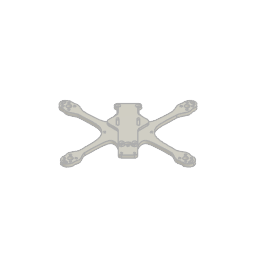
moineau (Autodesk Fusion 360 design; units mm, degrees)
Autodesk Fusion 360 part; units mm, degrees
sketch "Sketch1" plane through (0, 0, 0) normal (0, 0, 1) x (1, 0, 0)
  circle A0 centre (55.8574, 6.7392) radius 4.5 construction
  line L0 (55.8574, 6.7392) -> (52.6754, 9.9212) construction
  line L1 (219.6626, 222.0359) -> (219.6626, 222.0359)
  circle A1 centre (52.6754, 9.9212) radius 1.05
  circle A2 centre (55.8574, 6.7392) radius 2.25
  line L2 (42.8574, 9.2392) -> (42.8574, 4.2392) construction
  line L3 (55.8574, 6.7392) -> (61.4123, 6.7392) construction
  spline S0 degree 5 poles (64.6052, 6.7392) (64.6028, 6.815) (64.5921, 6.9823) (64.5587, 7.2805) (64.4799, 7.7571) (64.3247, 8.4054) (64.1108, 9.0216) (63.8323, 9.553) (63.4775, 10.0087) (63.0354, 10.4282) (62.4998, 10.855) (61.8755, 11.308) (61.1831, 11.7559) (60.4518, 12.1419) (59.713, 12.4068) (58.994, 12.5114) (58.3111, 12.462) (57.6641, 12.3267) (57.041, 12.1976) (56.421, 12.1615) (55.7776, 12.2677) (55.0823, 12.4938) (54.3087, 12.7668) (53.4369, 12.9885) (52.4575, 13.0608) (51.3775, 12.9063) (50.2215, 12.502) (49.011, 11.8911) (47.7686, 11.1568) (46.5151, 10.408) (45.2684, 9.7601) (44.2882, 9.4068) (43.567, 9.2696) (43.0928, 9.2392) (42.8574, 9.2392) knots 0 0 0 0 0 0 0.033333 0.066667 0.1 0.133333 0.166667 0.2 0.233333 0.266667 0.3 0.333333 0.366667 0.4 0.433333 0.466667 0.5 0.533333 0.566667 0.6 0.633333 0.666667 0.7 0.733333 0.766667 0.8 0.833333 0.866667 0.9 0.933333 0.966667 1 1 1 1 1 1
  line L4 (54.2959, 13.1912) -> (50.0454, 12.7812)
  line L5 (64.6536, 5.2576) -> (64.5569, 8.2208)
  line L6 (44.8576, 9.239) -> (40.8572, 9.2393)
  line L7 (0, 0) -> (70.7107, 70.7107) construction
  line L8 (-12.75, 12.75) -> (12.75, 12.75) construction
  line L9 (12.75, 12.75) -> (12.75, -12.75) construction
  line L10 (12.75, -12.75) -> (-12.75, -12.75) construction
  line L11 (-12.75, -12.75) -> (-12.75, 12.75) construction
  line L12 (12.75, -12.75) -> (-12.75, 12.75) construction
  circle A3 centre (12.75, 12.75) radius 1.05
  circle A4 centre (12.75, -12.75) radius 1.05
  line L13 (12.75, -12.75) -> (19.8211, -19.8211) construction
  line L14 (19.9636, -9.357) -> (25.1244, -14.5178)
  line L15 (12.75, 12.75) -> (14.9037, 12.0987) construction
  line L16 (12.75, 12.75) -> (15.3173, 13.1187) construction
  circle A5 centre (-12.75, 12.75) radius 1.05
  spline S1 degree 5 poles (60.9811, 6.7392) (60.9811, 6.886) (60.9796, 7.1794) (60.9724, 7.6186) (60.9623, 8.1894) (60.9925, 8.8095) (61.1129, 9.2564) (61.3477, 9.4734) (61.6899, 9.4412) (62.0445, 9.2424) (62.3497, 8.953) (62.5856, 8.6227) (62.7528, 8.2869) (62.8658, 7.964) (62.9398, 7.6579) (62.9854, 7.3611) (63.005, 7.1209) (63.0122, 6.9335) (63.0138, 6.8046) (63.0138, 6.7392) knots 0 0 0 0 0 0 0.066667 0.133333 0.2 0.266667 0.333333 0.4 0.466667 0.533333 0.6 0.666667 0.733333 0.8 0.866667 0.933333 1 1 1 1 1 1
  line L17 (60.9811, 5.9005) -> (60.9811, 7.5778)
  line L18 (61.2671, 9.4784) -> (61.9183, 9.3698)
  line L19 (63.0138, 7.3223) -> (63.0138, 6.1561)
  circle A6 centre (52.6754, 3.5572) radius 1.05
  circle A7 centre (59.0394, 3.5572) radius 1.05
  circle A8 centre (59.0394, 9.9212) radius 1.05
  circle A9 centre (23.3566, -16.2855) radius 1
  circle A10 centre (-12.75, 12.75) radius 1.05
  circle A11 centre (-12.75, 12.75) radius 1.05
  circle A12 centre (16.2855, -23.3566) radius 1
  circle A13 centre (12.75, -12.75) radius 1.05
  line L20 (9.357, -19.9636) -> (14.5178, -25.1244)
  line L21 (-12.75, 12.75) -> (-14.8713, 14.8713) construction
  line L22 (-20.3514, 9.3912) -> (-9.3912, 20.3514) construction
  circle A14 centre (-9.3912, 20.3514) radius 1.05
  circle A15 centre (-20.3514, 9.3912) radius 1.05
  line L23 (-19.114, 29.0135) -> (-29.0135, 19.114)
  line L24 (-12.75, 12.75) -> (-38.0129, 38.0129) construction
  line L25 (-19.114, 29.0135) -> (-17.1216, 29.1878)
  line L26 (-17.1216, 29.1878) -> (-11.2505, 23.3167)
  spline S2 degree 5 poles (-11.2505, 23.3167) (-11.2214, 23.2876) (-11.14, 23.2369) (-10.9486, 23.1834) (-10.5781, 23.1487) (-10.0185, 23.1302) (-9.5696, 23.1041) (-9.2669, 23.0627) (-9.0856, 23.0229) (-9, 23) knots 0 0 0 0 0 0 0.2 0.4 0.6 0.8 1 1 1 1 1 1
  line L27 (-11.5038, 23.57) -> (-10.9973, 23.0635)
  arc A16 (11.159, 11.1591) -> (11.1591, 11.1591) centre (10.8877, 13.3927) ccw
  arc A17 (-11.159, -11.1591) -> (-11.1591, -11.159) centre (-12.75, -12.75) ccw
  line L28 (-9.8162, 23.2188) -> (-8.1838, 22.7812)
  circle A18 centre (-12.75, -12.75) radius 1.05
  line L29 (-29.1878, 17.1216) -> (-23.3167, 11.2505)
  spline S3 degree 5 poles (-23.3167, 11.2505) (-23.2876, 11.2214) (-23.2369, 11.14) (-23.1834, 10.9486) (-23.1487, 10.5781) (-23.1302, 10.0185) (-23.1041, 9.5696) (-23.0627, 9.2669) (-23.0229, 9.0856) (-23, 9) knots 0 0 0 0 0 0 0.2 0.4 0.6 0.8 1 1 1 1 1 1
  line L30 (-23.57, 11.5038) -> (-23.0635, 10.9973)
  line L31 (-23.2188, 9.8162) -> (-22.7812, 8.1838)
  line L32 (-29.0135, 19.114) -> (-29.1878, 17.1216)
  line L33 (23.3566, -16.2855) -> (16.2855, -23.3566) construction
  line L34 (18.0533, -25.1244) -> (25.1244, -18.0533)
  arc A19 (14.5178, -25.1244) -> (18.0533, -25.1244) centre (16.2855, -23.3566) ccw
  arc A20 (18.0533, -21.5888) -> (17.6838, -21.2842) centre (16.2855, -23.3566) ccw construction
  arc A21 (21.2842, -17.6838) -> (21.5888, -18.0533) centre (23.3566, -16.2855) ccw construction
  arc A22 (25.1244, -18.0533) -> (25.1244, -14.5178) centre (23.3566, -16.2855) ccw
  line L35 (14.5345, -21.6048) -> (14.5054, -21.6339)
  line L36 (21.4731, -14.6417) -> (21.7061, -14.4078)
  circle A23 centre (55.8574, 6.7392) radius 37 construction
  spline S4 degree 5 poles (64.6052, 6.7392) (64.6028, 6.6634) (64.5921, 6.4961) (64.5587, 6.1979) (64.4799, 5.7213) (64.3247, 5.073) (64.1108, 4.4567) (63.8323, 3.9254) (63.4775, 3.4697) (63.0354, 3.0502) (62.4998, 2.6234) (61.8755, 2.1704) (61.1831, 1.7225) (60.4518, 1.3365) (59.713, 1.0715) (58.994, 0.967) (58.3111, 1.0163) (57.6641, 1.1517) (57.041, 1.2807) (56.421, 1.3168) (55.7776, 1.2106) (55.0823, 0.9846) (54.3087, 0.7116) (53.4369, 0.4899) (52.4575, 0.4175) (51.3775, 0.572) (50.2215, 0.9763) (49.011, 1.5872) (47.7686, 2.3215) (46.5151, 3.0704) (45.2684, 3.7183) (44.2882, 4.0715) (43.567, 4.2087) (43.0928, 4.2392) (42.8574, 4.2392) knots 0 0 0 0 0 0 0.033333 0.066667 0.1 0.133333 0.166667 0.2 0.233333 0.266667 0.3 0.333333 0.366667 0.4 0.433333 0.466667 0.5 0.533333 0.566667 0.6 0.633333 0.666667 0.7 0.733333 0.766667 0.8 0.833333 0.866667 0.9 0.933333 0.966667 1 1 1 1 1 1
  line L37 (64.6536, 8.2208) -> (64.5569, 5.2576)
  line L38 (54.2959, 0.2872) -> (50.0454, 0.6972)
  line L39 (44.8576, 4.2393) -> (40.8572, 4.239)
  circle A24 centre (55.8574, 6.7392) radius 34.5 construction
  circle A25 centre (12.75, 12.75) radius 2.25 construction
  spline S5 degree 5 poles (42.8574, 9.2392) (41.9558, 9.2392) (40.1768, 9.2381) (37.5805, 9.2331) (34.2689, 9.2281) (30.4157, 9.273) (26.8997, 9.4308) (23.7764, 9.7638) (21.0905, 10.3188) (18.8586, 11.1117) (17.0345, 12.0983) (15.8354, 12.979) (15.0487, 13.6574) (14.5694, 14.1126) (14.341, 14.341) knots 0 0 0 0 0 0 0.1 0.2 0.3 0.4 0.5 0.6 0.7 0.8 0.9 1 1 1 1 1 1
  line L40 (55.8574, 6.7392) -> (39.6365, 6.7392) construction
  spline S6 degree 5 poles (60.9811, 6.7392) (60.9811, 6.5924) (60.9796, 6.299) (60.9724, 5.8597) (60.9623, 5.2889) (60.9925, 4.6689) (61.1129, 4.2219) (61.3477, 4.005) (61.6899, 4.0372) (62.0445, 4.2359) (62.3497, 4.5254) (62.5856, 4.8556) (62.7528, 5.1915) (62.8658, 5.5144) (62.9398, 5.8204) (62.9854, 6.1172) (63.005, 6.3575) (63.0122, 6.5449) (63.0138, 6.6737) (63.0138, 6.7392) knots 0 0 0 0 0 0 0.066667 0.133333 0.2 0.266667 0.333333 0.4 0.466667 0.533333 0.6 0.666667 0.733333 0.8 0.866667 0.933333 1 1 1 1 1 1
  line L41 (60.9811, 7.5778) -> (60.9811, 5.9005)
  line L42 (61.2671, 4) -> (61.9183, 4.1085)
  line L43 (63.0138, 6.1561) -> (63.0138, 7.3223)
  spline S7 degree 5 poles (42.8574, 4.2392) (42.1901, 4.2392) (40.7827, 4.2297) (38.4535, 4.1868) (34.949, 4.0874) (30.1603, 3.9196) (25.3267, 3.7053) (20.9596, 3.2626) (17.5748, 2.3633) (16.0007, 0.1789) (16.3054, -3.2263) (17.5383, -6.132) (18.7041, -7.9522) (19.5348, -8.9282) (19.9636, -9.357) knots 0 0 0 0 0 0 0.1 0.2 0.3 0.4 0.5 0.6 0.7 0.8 0.9 1 1 1 1 1 1
  line L44 (17.5946, -6.988) -> (22.3327, -11.726)
  line L45 (20.6288, 3.4493) -> (16.141, 1.0742)
  line L46 (45.5972, 4.2392) -> (40.1176, 4.2392)
  line L47 (46.7254, 9.2392) -> (38.9894, 9.2392)
  line L48 (16.108, 12.574) -> (12.574, 16.108)
  spline S8 degree 5 poles (7.714, 65.3298) (7.7906, 65.3273) (7.96, 65.3164) (8.2624, 65.2825) (8.746, 65.2023) (9.4022, 65.0438) (10.0225, 64.8248) (10.5546, 64.5389) (11.0112, 64.1746) (11.4343, 63.721) (11.8689, 63.1728) (12.3303, 62.536) (12.7814, 61.8322) (13.161, 61.0907) (13.4086, 60.343) (13.4875, 59.6163) (13.4148, 58.9265) (13.2697, 58.2741) (13.1505, 57.6479) (13.1443, 57.0267) (13.2883, 56.3815) (13.5411, 55.6784) (13.8155, 54.884) (14.0063, 53.9733) (14.0189, 52.9331) (13.801, 51.7736) (13.3632, 50.5214) (12.7561, 49.2026) (12.06, 47.8463) (11.3703, 46.4802) (10.7848, 45.1298) (10.4695, 44.0785) (10.3475, 43.3128) (10.3204, 42.8131) (10.3204, 42.566) knots 0 0 0 0 0 0 0.033333 0.066667 0.1 0.133333 0.166667 0.2 0.233333 0.266667 0.3 0.333333 0.366667 0.4 0.433333 0.466667 0.5 0.533333 0.566667 0.6 0.633333 0.666667 0.7 0.733333 0.766667 0.8 0.833333 0.866667 0.9 0.933333 0.966667 1 1 1 1 1 1
  line L49 (6.2324, 65.3781) -> (9.1956, 65.2815)
  line L50 (14.166, 55.0205) -> (13.756, 50.7699)
  line L51 (10.3202, 44.5662) -> (10.3205, 40.5658)
  spline S9 degree 5 poles (10.3204, 42.566) (10.2984, 41.6849) (10.2471, 39.9441) (10.1481, 37.3965) (9.9851, 34.1337) (9.8047, 30.3201) (9.7427, 26.8287) (9.8943, 23.7216) (10.3307, 21.0485) (11.0771, 18.8293) (12.0702, 17.0176) (12.9709, 15.8271) (13.6578, 15.0453) (14.1136, 14.5684) (14.341, 14.341) knots 0 0 0 0 0 0 0.1 0.2 0.3 0.4 0.5 0.6 0.7 0.8 0.9 1 1 1 1 1 1
  line L52 (10.4158, 46.3946) -> (10.2249, 38.7374)
  line L53 (12.574, 16.108) -> (16.108, 12.574)
  spline S10 degree 5 poles (7.714, 65.3298) (7.6379, 65.3273) (7.4699, 65.3165) (7.1703, 65.2829) (6.6913, 65.2036) (6.0403, 65.0472) (5.4231, 64.8319) (4.8921, 64.5515) (4.4366, 64.194) (4.0159, 63.7481) (3.5857, 63.2077) (3.1282, 62.5782) (2.6776, 61.8809) (2.2929, 61.1458) (2.0346, 60.405) (1.9414, 59.6859) (2.0026, 59.0037) (2.1442, 58.3569) (2.2696, 57.7321) (2.2909, 57.1075) (2.1636, 56.4567) (1.9212, 55.753) (1.6464, 54.9716) (1.4414, 54.0926) (1.3992, 53.1039) (1.5722, 52.0042) (1.948, 50.8057) (2.4802, 49.531) (3.0957, 48.2088) (3.7082, 46.8708) (4.2293, 45.5482) (4.5103, 44.5237) (4.6191, 43.7829) (4.6432, 43.3022) (4.6432, 43.0652) knots 0 0 0 0 0 0 0.033333 0.066667 0.1 0.133333 0.166667 0.2 0.233333 0.266667 0.3 0.333333 0.366667 0.4 0.433333 0.466667 0.5 0.533333 0.566667 0.6 0.633333 0.666667 0.7 0.733333 0.766667 0.8 0.833333 0.866667 0.9 0.933333 0.966667 1 1 1 1 1 1
  line L54 (9.1956, 65.3781) -> (6.2324, 65.2815)
  line L55 (1.262, 55.0205) -> (1.672, 50.7699)
  line L56 (4.6433, 45.0654) -> (4.643, 41.065)
  circle A26 centre (4.532, 53.4) radius 1.05
  circle A27 centre (10.896, 53.4) radius 1.05
  circle A28 centre (7.714, 56.582) radius 2.25
  circle A29 centre (10.896, 59.7639) radius 1.05
  circle A30 centre (4.532, 59.7639) radius 1.05
  spline S11 degree 5 poles (7.714, 61.7057) (7.5672, 61.7057) (7.2738, 61.7041) (6.8346, 61.697) (6.2637, 61.6869) (5.6437, 61.7171) (5.1968, 61.8375) (4.9798, 62.0722) (5.012, 62.4145) (5.2108, 62.769) (5.5002, 63.0742) (5.8305, 63.3102) (6.1663, 63.4774) (6.4892, 63.5904) (6.7952, 63.6644) (7.0921, 63.7099) (7.3323, 63.7296) (7.5197, 63.7368) (7.6486, 63.7384) (7.714, 63.7384) knots 0 0 0 0 0 0 0.066667 0.133333 0.2 0.266667 0.333333 0.4 0.466667 0.533333 0.6 0.666667 0.733333 0.8 0.866667 0.933333 1 1 1 1 1 1
  line L57 (8.5526, 61.7057) -> (6.8754, 61.7057)
  line L58 (4.9748, 61.9917) -> (5.0833, 62.6429)
  line L59 (7.1309, 63.7384) -> (8.2971, 63.7384)
  spline S12 degree 5 poles (7.714, 61.7057) (7.8608, 61.7057) (8.1542, 61.7041) (8.5935, 61.697) (9.1643, 61.6869) (9.7843, 61.7171) (10.2312, 61.8375) (10.4482, 62.0722) (10.416, 62.4145) (10.2172, 62.769) (9.9278, 63.0742) (9.5975, 63.3102) (9.2617, 63.4774) (8.9388, 63.5904) (8.6328, 63.6644) (8.3359, 63.7099) (8.0957, 63.7296) (7.9083, 63.7368) (7.7794, 63.7384) (7.714, 63.7384) knots 0 0 0 0 0 0 0.066667 0.133333 0.2 0.266667 0.333333 0.4 0.466667 0.533333 0.6 0.666667 0.733333 0.8 0.866667 0.933333 1 1 1 1 1 1
  line L60 (6.8754, 61.7057) -> (8.5526, 61.7057)
  line L61 (10.4532, 61.9917) -> (10.3447, 62.6429)
  line L62 (8.2971, 63.7384) -> (7.1309, 63.7384)
  spline S13 degree 5 poles (4.6432, 43.0652) (4.6723, 42.2697) (4.7118, 40.6946) (4.7144, 38.3799) (4.616, 35.3633) (4.3554, 31.6334) (3.9642, 27.9249) (3.3555, 24.4479) (2.3651, 21.5867) (0.5507, 20.4458) (-2.1027, 20.8951) (-4.7107, 21.8641) (-6.8153, 22.5185) (-8.2642, 22.856) (-9, 23) knots 0 0 0 0 0 0 0.1 0.2 0.3 0.4 0.5 0.6 0.7 0.8 0.9 1 1 1 1 1 1
  line L63 (-4.4613, 22.1117) -> (-13.5387, 23.8883)
  line L64 (3.6977, 25.0349) -> (1.5288, 20.5164)
  spline S14 degree 5 poles (-6.7392, -64.6052) (-6.815, -64.6028) (-6.9823, -64.5921) (-7.2805, -64.5587) (-7.7571, -64.4799) (-8.4054, -64.3247) (-9.0216, -64.1108) (-9.553, -63.8323) (-10.0087, -63.4775) (-10.4282, -63.0354) (-10.855, -62.4998) (-11.308, -61.8755) (-11.7559, -61.1831) (-12.1419, -60.4518) (-12.4068, -59.713) (-12.5114, -58.994) (-12.462, -58.3111) (-12.3267, -57.6641) (-12.1976, -57.041) (-12.1615, -56.421) (-12.2677, -55.7776) (-12.4938, -55.0823) (-12.7668, -54.3087) (-12.9885, -53.4369) (-13.0608, -52.4575) (-12.9063, -51.3775) (-12.502, -50.2215) (-11.8911, -49.011) (-11.1568, -47.7686) (-10.408, -46.5151) (-9.7601, -45.2684) (-9.4068, -44.2882) (-9.2696, -43.567) (-9.2392, -43.0928) (-9.2392, -42.8574) knots 0 0 0 0 0 0 0.033333 0.066667 0.1 0.133333 0.166667 0.2 0.233333 0.266667 0.3 0.333333 0.366667 0.4 0.433333 0.466667 0.5 0.533333 0.566667 0.6 0.633333 0.666667 0.7 0.733333 0.766667 0.8 0.833333 0.866667 0.9 0.933333 0.966667 1 1 1 1 1 1
  line L65 (-5.2576, -64.6536) -> (-8.2208, -64.5569)
  line L66 (-13.1912, -54.2959) -> (-12.7812, -50.0454)
  line L67 (-9.239, -44.8576) -> (-9.2393, -40.8572)
  spline S15 degree 5 poles (-9.2392, -42.8574) (-9.2392, -41.9558) (-9.2381, -40.1768) (-9.2331, -37.5805) (-9.2281, -34.2689) (-9.273, -30.4157) (-9.4308, -26.8997) (-9.7638, -23.7764) (-10.3188, -21.0905) (-11.1117, -18.8586) (-12.0983, -17.0345) (-12.979, -15.8354) (-13.6574, -15.0487) (-14.1126, -14.5694) (-14.341, -14.341) knots 0 0 0 0 0 0 0.1 0.2 0.3 0.4 0.5 0.6 0.7 0.8 0.9 1 1 1 1 1 1
  line L68 (-9.2392, -46.7254) -> (-9.2392, -38.9894)
  line L69 (-12.574, -16.108) -> (-16.108, -12.574)
  spline S16 degree 5 poles (-6.7392, -64.6052) (-6.6634, -64.6028) (-6.4961, -64.5921) (-6.1979, -64.5587) (-5.7213, -64.4799) (-5.073, -64.3247) (-4.4567, -64.1108) (-3.9254, -63.8323) (-3.4697, -63.4775) (-3.0502, -63.0354) (-2.6234, -62.4998) (-2.1704, -61.8755) (-1.7225, -61.1831) (-1.3365, -60.4518) (-1.0715, -59.713) (-0.967, -58.994) (-1.0163, -58.3111) (-1.1517, -57.6641) (-1.2807, -57.041) (-1.3168, -56.421) (-1.2106, -55.7776) (-0.9846, -55.0823) (-0.7116, -54.3087) (-0.4899, -53.4369) (-0.4175, -52.4575) (-0.572, -51.3775) (-0.9763, -50.2215) (-1.5872, -49.011) (-2.3215, -47.7686) (-3.0704, -46.5151) (-3.7183, -45.2684) (-4.0715, -44.2882) (-4.2087, -43.567) (-4.2392, -43.0928) (-4.2392, -42.8574) knots 0 0 0 0 0 0 0.033333 0.066667 0.1 0.133333 0.166667 0.2 0.233333 0.266667 0.3 0.333333 0.366667 0.4 0.433333 0.466667 0.5 0.533333 0.566667 0.6 0.633333 0.666667 0.7 0.733333 0.766667 0.8 0.833333 0.866667 0.9 0.933333 0.966667 1 1 1 1 1 1
  line L70 (-8.2208, -64.6536) -> (-5.2576, -64.5569)
  line L71 (-0.2872, -54.2959) -> (-0.6972, -50.0454)
  line L72 (-4.2393, -44.8576) -> (-4.239, -40.8572)
  spline S17 degree 5 poles (-4.2392, -42.8574) (-4.2392, -42.1901) (-4.2297, -40.7827) (-4.1868, -38.4535) (-4.0874, -34.949) (-3.9196, -30.1603) (-3.7053, -25.3267) (-3.2626, -20.9596) (-2.3633, -17.5748) (-0.1789, -16.0007) (3.2263, -16.3054) (6.132, -17.5383) (7.9522, -18.7041) (8.9282, -19.5348) (9.357, -19.9636) knots 0 0 0 0 0 0 0.1 0.2 0.3 0.4 0.5 0.6 0.7 0.8 0.9 1 1 1 1 1 1
  line L73 (-4.2392, -45.5972) -> (-4.2392, -40.1176)
  line L74 (-3.4493, -20.6288) -> (-1.0742, -16.141)
  line L75 (6.988, -17.5946) -> (11.726, -22.3327)
  circle A31 centre (-3.5572, -52.6754) radius 1.05
  circle A32 centre (-6.7392, -55.8574) radius 2.25
  circle A33 centre (-9.9212, -52.6754) radius 1.05
  circle A34 centre (-9.9212, -59.0394) radius 1.05
  circle A35 centre (-3.5572, -59.0394) radius 1.05
  spline S18 degree 5 poles (-6.7392, -60.9811) (-6.5924, -60.9811) (-6.299, -60.9796) (-5.8597, -60.9724) (-5.2889, -60.9623) (-4.6689, -60.9925) (-4.2219, -61.1129) (-4.005, -61.3477) (-4.0372, -61.6899) (-4.2359, -62.0445) (-4.5254, -62.3497) (-4.8556, -62.5856) (-5.1915, -62.7528) (-5.5144, -62.8658) (-5.8204, -62.9398) (-6.1172, -62.9854) (-6.3575, -63.005) (-6.5449, -63.0122) (-6.6737, -63.0138) (-6.7392, -63.0138) knots 0 0 0 0 0 0 0.066667 0.133333 0.2 0.266667 0.333333 0.4 0.466667 0.533333 0.6 0.666667 0.733333 0.8 0.866667 0.933333 1 1 1 1 1 1
  line L76 (-7.5778, -60.9811) -> (-5.9005, -60.9811)
  line L77 (-4, -61.2671) -> (-4.1085, -61.9183)
  line L78 (-6.1561, -63.0138) -> (-7.3223, -63.0138)
  spline S19 degree 5 poles (-6.7392, -60.9811) (-6.886, -60.9811) (-7.1794, -60.9796) (-7.6186, -60.9724) (-8.1894, -60.9623) (-8.8095, -60.9925) (-9.2564, -61.1129) (-9.4734, -61.3477) (-9.4412, -61.6899) (-9.2424, -62.0445) (-8.953, -62.3497) (-8.6227, -62.5856) (-8.2869, -62.7528) (-7.964, -62.8658) (-7.6579, -62.9398) (-7.3611, -62.9854) (-7.1209, -63.005) (-6.9335, -63.0122) (-6.8046, -63.0138) (-6.7392, -63.0138) knots 0 0 0 0 0 0 0.066667 0.133333 0.2 0.266667 0.333333 0.4 0.466667 0.533333 0.6 0.666667 0.733333 0.8 0.866667 0.933333 1 1 1 1 1 1
  line L79 (-5.9005, -60.9811) -> (-7.5778, -60.9811)
  line L80 (-9.4784, -61.2671) -> (-9.3698, -61.9183)
  line L81 (-7.3223, -63.0138) -> (-6.1561, -63.0138)
  line L82 (4.5096, 46.7096) -> (4.7768, 39.4209)
  circle A36 centre (12.75, -12.75) radius 2.25 construction
  line L83 (14.341, -11.159) -> (11.159, -14.341) construction
  arc A37 (10.7701, -3.699) -> (8.6488, -3.699) centre (9.7094, -4.7597) ccw
  line L84 (8.6488, -3.699) -> (3.699, -8.6488)
  arc A38 (3.699, -8.6488) -> (3.699, -10.7701) centre (4.7597, -9.7094) ccw
  line L85 (3.699, -10.7701) -> (6.5275, -13.5985)
  arc A39 (6.5275, -13.5985) -> (8.6488, -13.5985) centre (7.5881, -12.5379) ccw
  line L86 (8.6488, -13.5985) -> (13.5985, -8.6488)
  arc A40 (13.5985, -8.6488) -> (13.5985, -6.5275) centre (12.5379, -7.5881) ccw
  line L87 (13.5985, -6.5275) -> (10.7701, -3.699)
  circle A41 centre (7.714, 56.582) radius 34.5 construction
  circle A42 centre (7.714, 56.582) radius 37 construction
  spline S20 degree 5 poles (-65.3298, -7.714) (-65.3273, -7.7906) (-65.3164, -7.96) (-65.2825, -8.2624) (-65.2023, -8.746) (-65.0438, -9.4022) (-64.8248, -10.0225) (-64.5389, -10.5546) (-64.1746, -11.0112) (-63.721, -11.4343) (-63.1728, -11.8689) (-62.536, -12.3303) (-61.8322, -12.7814) (-61.0907, -13.161) (-60.343, -13.4086) (-59.6163, -13.4875) (-58.9265, -13.4148) (-58.2741, -13.2697) (-57.6479, -13.1505) (-57.0267, -13.1443) (-56.3815, -13.2883) (-55.6784, -13.5411) (-54.884, -13.8155) (-53.9733, -14.0063) (-52.9331, -14.0189) (-51.7736, -13.801) (-50.5214, -13.3632) (-49.2026, -12.7561) (-47.8463, -12.06) (-46.4802, -11.3703) (-45.1298, -10.7848) (-44.0785, -10.4695) (-43.3128, -10.3475) (-42.8131, -10.3204) (-42.566, -10.3204) knots 0 0 0 0 0 0 0.033333 0.066667 0.1 0.133333 0.166667 0.2 0.233333 0.266667 0.3 0.333333 0.366667 0.4 0.433333 0.466667 0.5 0.533333 0.566667 0.6 0.633333 0.666667 0.7 0.733333 0.766667 0.8 0.833333 0.866667 0.9 0.933333 0.966667 1 1 1 1 1 1
  line L88 (-65.3781, -6.2324) -> (-65.2815, -9.1956)
  line L89 (-55.0205, -14.166) -> (-50.7699, -13.756)
  line L90 (-44.5662, -10.3202) -> (-40.5658, -10.3205)
  spline S21 degree 5 poles (-42.566, -10.3204) (-41.6849, -10.2984) (-39.9441, -10.2471) (-37.3965, -10.1481) (-34.1337, -9.9851) (-30.3201, -9.8047) (-26.8287, -9.7427) (-23.7216, -9.8943) (-21.0485, -10.3307) (-18.8293, -11.0771) (-17.0176, -12.0702) (-15.8271, -12.9709) (-15.0453, -13.6578) (-14.5684, -14.1136) (-14.341, -14.341) knots 0 0 0 0 0 0 0.1 0.2 0.3 0.4 0.5 0.6 0.7 0.8 0.9 1 1 1 1 1 1
  line L91 (-46.3946, -10.4158) -> (-38.7374, -10.2249)
  line L92 (-16.108, -12.574) -> (-12.574, -16.108)
  spline S22 degree 5 poles (-65.3298, -7.714) (-65.3273, -7.6379) (-65.3165, -7.4699) (-65.2829, -7.1703) (-65.2036, -6.6913) (-65.0472, -6.0403) (-64.8319, -5.4231) (-64.5515, -4.8921) (-64.194, -4.4366) (-63.7481, -4.0159) (-63.2077, -3.5857) (-62.5782, -3.1282) (-61.8809, -2.6776) (-61.1458, -2.2929) (-60.405, -2.0346) (-59.6859, -1.9414) (-59.0037, -2.0026) (-58.3569, -2.1442) (-57.7321, -2.2696) (-57.1075, -2.2909) (-56.4567, -2.1636) (-55.753, -1.9212) (-54.9716, -1.6464) (-54.0926, -1.4414) (-53.1039, -1.3992) (-52.0042, -1.5722) (-50.8057, -1.948) (-49.531, -2.4802) (-48.2088, -3.0957) (-46.8708, -3.7082) (-45.5482, -4.2293) (-44.5237, -4.5103) (-43.7829, -4.6191) (-43.3022, -4.6432) (-43.0652, -4.6432) knots 0 0 0 0 0 0 0.033333 0.066667 0.1 0.133333 0.166667 0.2 0.233333 0.266667 0.3 0.333333 0.366667 0.4 0.433333 0.466667 0.5 0.533333 0.566667 0.6 0.633333 0.666667 0.7 0.733333 0.766667 0.8 0.833333 0.866667 0.9 0.933333 0.966667 1 1 1 1 1 1
  line L93 (-65.3781, -9.1956) -> (-65.2815, -6.2324)
  line L94 (-55.0205, -1.262) -> (-50.7699, -1.672)
  line L95 (-45.0654, -4.6433) -> (-41.065, -4.643)
  spline S23 degree 5 poles (-23.3167, 11.2505) (-23.2876, 11.2214) (-23.2369, 11.14) (-23.1834, 10.9486) (-23.1487, 10.5781) (-23.1302, 10.0185) (-23.1041, 9.5696) (-23.0627, 9.2669) (-23.0229, 9.0856) (-23, 9) knots 0 0 0 0 0 0 0.2 0.4 0.6 0.8 1 1 1 1 1 1
  line L96 (-23.57, 11.5038) -> (-23.0635, 10.9973)
  line L97 (-23.2188, 9.8162) -> (-22.7812, 8.1838)
  line L98 (-29.1878, 17.1216) -> (-23.3167, 11.2505)
  line L99 (-29.0135, 19.114) -> (-29.1878, 17.1216)
  line L100 (-29.0135, 19.114) -> (-19.114, 29.0135)
  spline S24 degree 5 poles (-43.0652, -4.6432) (-42.2697, -4.6723) (-40.6946, -4.7118) (-38.3799, -4.7144) (-35.3633, -4.616) (-31.6334, -4.3554) (-27.9249, -3.9642) (-24.4479, -3.3555) (-21.5867, -2.3651) (-20.4458, -0.5507) (-20.8951, 2.1027) (-21.8641, 4.7107) (-22.5185, 6.8153) (-22.856, 8.2642) (-23, 9) knots 0 0 0 0 0 0 0.1 0.2 0.3 0.4 0.5 0.6 0.7 0.8 0.9 1 1 1 1 1 1
  line L101 (-46.7096, -4.5096) -> (-39.4209, -4.7768)
  line L102 (-25.0349, -3.6977) -> (-20.5164, -1.5288)
  line L103 (-22.1117, 4.4613) -> (-23.8883, 13.5387)
  circle A43 centre (-53.4, -4.532) radius 1.05
  circle A44 centre (-56.582, -7.714) radius 2.25
  circle A45 centre (-59.7639, -4.532) radius 1.05
  circle A46 centre (-53.4, -10.896) radius 1.05
  circle A47 centre (-59.7639, -10.896) radius 1.05
  spline S25 degree 5 poles (-61.7057, -7.714) (-61.7057, -7.8608) (-61.7041, -8.1542) (-61.697, -8.5935) (-61.6869, -9.1643) (-61.7171, -9.7843) (-61.8375, -10.2312) (-62.0722, -10.4482) (-62.4145, -10.416) (-62.769, -10.2172) (-63.0742, -9.9278) (-63.3102, -9.5975) (-63.4774, -9.2617) (-63.5904, -8.9388) (-63.6644, -8.6328) (-63.7099, -8.3359) (-63.7296, -8.0957) (-63.7368, -7.9083) (-63.7384, -7.7794) (-63.7384, -7.714) knots 0 0 0 0 0 0 0.066667 0.133333 0.2 0.266667 0.333333 0.4 0.466667 0.533333 0.6 0.666667 0.733333 0.8 0.866667 0.933333 1 1 1 1 1 1
  line L104 (-61.7057, -6.8754) -> (-61.7057, -8.5526)
  line L105 (-61.9917, -10.4532) -> (-62.6429, -10.3447)
  line L106 (-63.7384, -8.2971) -> (-63.7384, -7.1309)
  spline S26 degree 5 poles (-61.7057, -7.714) (-61.7057, -7.5672) (-61.7041, -7.2738) (-61.697, -6.8346) (-61.6869, -6.2637) (-61.7171, -5.6437) (-61.8375, -5.1968) (-62.0722, -4.9798) (-62.4145, -5.012) (-62.769, -5.2108) (-63.0742, -5.5002) (-63.3102, -5.8305) (-63.4774, -6.1663) (-63.5904, -6.4892) (-63.6644, -6.7952) (-63.7099, -7.0921) (-63.7296, -7.3323) (-63.7368, -7.5197) (-63.7384, -7.6486) (-63.7384, -7.714) knots 0 0 0 0 0 0 0.066667 0.133333 0.2 0.266667 0.333333 0.4 0.466667 0.533333 0.6 0.666667 0.733333 0.8 0.866667 0.933333 1 1 1 1 1 1
  line L107 (-61.7057, -8.5526) -> (-61.7057, -6.8754)
  line L108 (-61.9917, -4.9748) -> (-62.6429, -5.0833)
  line L109 (-63.7384, -7.1309) -> (-63.7384, -8.2971)
  point P0 (64.123, 8.9336)
  point P1 (62.5074, 10.8385)
  point P2 (59.1274, 12.4657)
  point P3 (56.3632, 12.1999)
  point P4 (52.1707, 12.9862)
  point P5 (42.8574, 6.7392)
  point P6 (26.4716, -15.865)
  point P7 (19.8211, -19.8211)
  point P8 (61.5927, 9.4241)
  point P9 (62.8098, 8.1097)
  point P10 (-14.8713, 14.8713)
  point P11 (-24.0637, 24.0637)
  point P12 (19.8211, -19.8211)
  point P13 (12.016, 12.016)
  point P14 (64.123, 4.5448)
  point P15 (62.5074, 2.6399)
  point P16 (59.1274, 1.0127)
  point P17 (56.3632, 1.2785)
  point P18 (52.1707, 0.4922)
  point P19 (20.5999, 10.5538)
  point P20 (61.5927, 4.0543)
  point P21 (62.8098, 5.3687)
  point P22 (18.3849, 2.2618)
  point P23 (9.9084, 64.8475)
  point P24 (11.8133, 63.232)
  point P25 (13.4405, 59.852)
  point P26 (13.1747, 57.0877)
  point P27 (13.961, 52.8952)
  point P28 (10.5538, 20.5999)
  point P29 (5.5196, 64.8475)
  point P30 (3.6147, 63.232)
  point P31 (1.9875, 59.852)
  point P32 (2.2533, 57.0877)
  point P33 (1.467, 52.8952)
  point P34 (5.0291, 62.3173)
  point P35 (6.3435, 63.5343)
  point P36 (10.3989, 62.3173)
  point P37 (9.0845, 63.5343)
  point P38 (2.6132, 22.7757)
  point P39 (-8.9336, -64.123)
  point P40 (-10.8385, -62.5074)
  point P41 (-12.4657, -59.1274)
  point P42 (-12.1999, -56.3632)
  point P43 (-12.9862, -52.1707)
  point P44 (-10.5538, -20.5999)
  point P45 (-4.5448, -64.123)
  point P46 (-2.6399, -62.5074)
  point P47 (-1.0127, -59.1274)
  point P48 (-1.2785, -56.3632)
  point P49 (-0.4922, -52.1707)
  point P50 (-2.2618, -18.3849)
  point P51 (-4.0543, -61.5927)
  point P52 (-5.3687, -62.8098)
  point P53 (-9.4241, -61.5927)
  point P54 (-8.1097, -62.8098)
  point P55 (-64.8475, -9.9084)
  point P56 (-63.232, -11.8133)
  point P57 (-59.852, -13.4405)
  point P58 (-57.0877, -13.1747)
  point P59 (-52.8952, -13.961)
  point P60 (-20.5999, -10.5538)
  point P61 (-64.8475, -5.5196)
  point P62 (-63.232, -3.6147)
  point P63 (-59.852, -1.9875)
  point P64 (-57.0877, -2.2533)
  point P65 (-52.8952, -1.467)
  point P66 (-22.7757, -2.6132)
  point P67 (-62.3173, -10.3989)
  point P68 (-63.5343, -9.0845)
  point P69 (-62.3173, -5.0291)
  point P70 (-63.5343, -6.3435)
  dimension "d1" = 9
  dimension "d19" = 5
  dimension "d20" = 25.5
  dimension "d21" = 25.5
  dimension "d22" = 2.1
  dimension "d24" = 4.5
  dimension "d25" = 2.1
  dimension "d26" = 10
  dimension "d28" = 25
  dimension "d31" = 360
  dimension "d32" = 2.1
  dimension "d35" = 2.5
  dimension "d44" = 2
  dimension "d45" = 3
  dimension "d46" = 15.5
  dimension "d47" = 2.1
  dimension "d48" = 2.1
  dimension "d49" = 14
  dimension "d50" = 13
  dimension "d51" = 2
  dimension "d52" = 140
  dimension "d53" = 3.5
  dimension "d76" = 13
  dimension "d191" = 74
  dimension "d192" = 69
  dimension "d193" = 4.5
  dimension "d208" = 69
  dimension "d209" = 74
  dimension "d218" = 10
  dimension "d219" = 2.5
  constraint coincident L7.start origin
  constraint coincident A0.centre L0.start
  constraint coincident A0 L0.end
  constraint coincident L0.end A1.centre
  constraint coincident L3 S0.start
  constraint midpoint P4 L4
  constraint midpoint S0.start L5
  constraint midpoint L2.start L6
  constraint coincident L8.end L9.start
  constraint coincident L9.end L10.start
  constraint coincident P12 P7
  constraint midpoint L2 P5
  constraint coincident P6 L14
  constraint tangent L14 A21
  constraint coincident L3 S1.end
  constraint coincident L3 S1.start
  constraint parallel L12 L14
  constraint concentric A9 A21
  constraint symmetric L7 A4 A10
  constraint symmetric L12 A4 A13
  constraint symmetric L12 L14.start L20.start
  constraint symmetric L12 A21.start A20.end
  constraint symmetric L12 L14.end L20.end
  constraint symmetric L12 A19 A21
  constraint symmetric L12 A9 A12
  constraint symmetric L12 A10 A11
  constraint coincident L8.start L11.end
  constraint parallel L12 L21
  constraint perpendicular L12 L22
  constraint midpoint L22 P10
  constraint coincident P10 L21.end
  constraint coincident L22.end A14.centre
  constraint coincident L22.start A15.centre
  constraint parallel L22 L23
  constraint midpoint L23 P11
  constraint parallel L21 L24
  constraint coincident P11 L24
  constraint parallel L24 L26
  constraint midpoint L26.end L27
  constraint parallel L26 L27
  constraint midpoint S2.end L28
  constraint symmetric L12 A3 A18
  constraint symmetric L12 L23.start L23.end
  constraint symmetric L12 L25.end L29.start
  constraint symmetric L12 L26.end L29.end
  constraint symmetric L12 S2.end S3.end
  constraint symmetric L12 L27.start L30.start
  constraint symmetric L12 L27.end L30.end
  constraint symmetric L12 L28.start L31.start
  constraint symmetric L12 L28.end L31.end
  constraint coincident A9.centre L33.start
  constraint coincident A12.centre L33.end
  constraint perpendicular L13 L33
  constraint midpoint L33 P12
  constraint coincident L33 A20.start
  constraint concentric A19 A20
  constraint coincident L33 A21.end
  constraint concentric A21 A22
  constraint coincident L34.end A21
  constraint coincident A21 L36.start
  constraint collinear L35 L36
  constraint coincident A21 L36.end
  constraint symmetric L2.start L3 L2.end
  constraint symmetric L3 S0.start S4.start
  constraint symmetric L3 P0 P14
  constraint symmetric L3 P1 P15
  constraint symmetric L3 P2 P16
  constraint symmetric L3 P3 P17
  constraint symmetric L3 P4 P18
  constraint symmetric L3 L4.start L38.start
  constraint symmetric L3 L4.end L38.end
  constraint symmetric L3 L5.start L37.start
  constraint symmetric L3 L5.end L37.end
  constraint symmetric L3 L6.start L39.start
  constraint symmetric L3 L6.end L39.end
  constraint concentric A2 A24
  constraint coincident L15.end A25
  constraint coincident A25 S5.end
  constraint coincident L7 S5.end
  constraint parallel L3 L40
  constraint vertical L2
  constraint coincident P5 L40
  constraint symmetric L3 S1.start S6.start
  constraint symmetric L3 P8 P20
  constraint symmetric L3 P9 P21
  constraint symmetric L3 S1.end S6.end
  constraint symmetric L3 L17.start L17.end
  constraint symmetric L3 L17.end L17.start
  constraint symmetric L3 L18.start L42.start
  constraint symmetric L3 L18.end L42.end
  constraint symmetric L3 L19.start L19.end
  constraint symmetric L3 L19.end L19.start
  constraint midpoint L14.start L44
  constraint coincident L14 L44.end
  constraint midpoint P22 L45
  constraint midpoint L2.end L46
  constraint perpendicular L2 L46
  constraint midpoint L2.start L47
  constraint perpendicular L2 L47
  constraint midpoint S5.end L48
  constraint perpendicular L7 L48
  constraint coincident L8 L9.start
  constraint symmetric L7 P19 P28
  constraint symmetric L7 S5.end S9.end
  constraint symmetric L7 L48.start L48.end
  constraint symmetric L7 L48.end L48.start
  constraint midpoint S2.end L63
  constraint midpoint P38 L64
  constraint midpoint S10.end L82
  constraint symmetric L2.start L12 S14.end
  constraint symmetric L2.end L12 S16.end
  constraint symmetric A1 L12 A33
  constraint symmetric A2 L12 A32
  constraint symmetric S0.start L12 S14.start
  constraint symmetric P0 L12 P39
  constraint symmetric P1 L12 P40
  constraint symmetric P2 L12 P41
  constraint symmetric P3 L12 P42
  constraint symmetric P4 L12 P43
  constraint symmetric L4.start L12 L66.start
  constraint symmetric L4.end L12 L66.end
  constraint symmetric L5.start L12 L65.start
  constraint symmetric L5.end L12 L65.end
  constraint symmetric L6.start L12 L67.start
  constraint symmetric L6.end L12 L67.end
  constraint symmetric L12 S1.start S18.start
  constraint symmetric L12 P8 P53
  constraint symmetric L12 P9 P54
  constraint symmetric L12 S1.end S18.end
  constraint symmetric L12 L17.start L76.end
  constraint symmetric L12 L17.end L76.start
  constraint symmetric L12 L18.start L80.start
  constraint symmetric L12 L18.end L80.end
  constraint symmetric L12 L19.start L78.end
  constraint symmetric L12 L19.end L78.start
  constraint symmetric L12 A6 A31
  constraint symmetric L12 A7 A35
  constraint symmetric L12 A8 A34
  constraint symmetric L12 S0.start S14.start
  constraint symmetric L12 P14 P45
  constraint symmetric L12 P15 P46
  constraint symmetric L12 P16 P47
  constraint symmetric L12 P17 P48
  constraint symmetric L12 P18 P49
  constraint symmetric L12 L2.end S16.end
  constraint symmetric L12 L37.start L70.start
  constraint symmetric L12 L37.end L70.end
  constraint symmetric L12 L38.start L71.start
  constraint symmetric L12 L38.end L71.end
  constraint symmetric L12 L39.start L72.start
  constraint symmetric L12 L39.end L72.end
  constraint symmetric L12 P19 P44
  constraint symmetric L12 S5.end S15.end
  constraint symmetric L12 P20 P51
  constraint symmetric L12 P21 P52
  constraint symmetric L12 L42.start L77.start
  constraint symmetric L12 L42.end L77.end
  constraint symmetric L12 P22 P50
  constraint symmetric L12 L44.start L75.start
  constraint symmetric L12 L44.end L75.end
  constraint symmetric L12 L45.start L74.start
  constraint symmetric L12 L45.end L74.end
  constraint symmetric L12 L46.start L73.start
  constraint symmetric L12 L46.end L73.end
  constraint symmetric L12 L47.start L68.start
  constraint symmetric L12 L47.end L68.end
  constraint symmetric L12 L48.start L69.start
  constraint symmetric L12 L48.end L69.end
  constraint coincident A36 L83.start
  constraint coincident A36 L83.end
  constraint coincident L9.end L83
  constraint perpendicular L12 L83
  constraint concentric A28 A41
  constraint concentric A41 A42
  constraint midpoint S10.end L56
  constraint symmetric L12 L23.end L23.start
  constraint symmetric L12 S8.start S20.start
  constraint symmetric L12 P23 P55
  constraint symmetric L12 P24 P56
  constraint symmetric L12 P25 P57
  constraint symmetric L12 P26 P58
  constraint symmetric L12 P27 P59
  constraint symmetric L12 S8.end S20.end
  constraint symmetric L12 L49.start L88.start
  constraint symmetric L12 L49.end L88.end
  constraint symmetric L12 L50.start L89.start
  constraint symmetric L12 L50.end L89.end
  constraint symmetric L12 L51.start L90.start
  constraint symmetric L12 L51.end L90.end
  constraint symmetric L12 P28 P60
  constraint symmetric L12 L52.start L91.start
  constraint symmetric L12 L52.end L91.end
  constraint symmetric L12 P29 P61
  constraint symmetric L12 P30 P62
  constraint symmetric L12 P31 P63
  constraint symmetric L12 P32 P64
  constraint symmetric L12 P33 P65
  constraint symmetric L12 S10.end S22.end
  constraint symmetric L12 L54.start L93.start
  constraint symmetric L12 L54.end L93.end
  constraint symmetric L12 L55.start L94.start
  constraint symmetric L12 L55.end L94.end
  constraint symmetric L12 L56.start L95.start
  constraint symmetric L12 L56.end L95.end
  constraint symmetric L12 A26 A43
  constraint symmetric L12 A27 A46
  constraint symmetric L12 A28 A44
  constraint symmetric L12 A29 A47
  constraint symmetric L12 A30 A45
  constraint symmetric L12 S11.start S25.start
  constraint symmetric L12 P34 P69
  constraint symmetric L12 P35 P70
  constraint symmetric L12 S11.end S25.end
  constraint symmetric L12 L57.start L104.end
  constraint symmetric L12 L57.end L104.start
  constraint symmetric L12 L58.start L108.start
  constraint symmetric L12 L58.end L108.end
  constraint symmetric L12 L59.start L106.end
  constraint symmetric L12 L59.end L106.start
  constraint symmetric L12 P36 P67
  constraint symmetric L12 P37 P68
  constraint symmetric L12 L61.start L105.start
  constraint symmetric L12 L61.end L105.end
  constraint symmetric L12 P38 P66
  constraint symmetric L12 L63.start L103.start
  constraint symmetric L12 L63.end L103.end
  constraint symmetric L12 L64.start L102.start
  constraint symmetric L12 L64.end L102.end
  constraint symmetric L12 L82.start L101.start
  constraint symmetric L12 L82.end L101.end
  constraint parallel L33 L34
  measures "d1" diameter of A0
  measures "d19" distance of L2.start L2.end
  measures "d20" distance of L8.start L8.end
  measures "d21" distance of L8.start L10.end
  measures "d22" diameter of A3
  measures "d24" diameter of A16
  measures "d25" diameter of A4
  measures "d26" distance of L9.end P12
  measures "d28" angle of L15 L16
  measures "d32" diameter of A1
  measures "d35" radius of A21
  measures "d44" diameter of A9
  measures "d45" distance of L8.start P10
  measures "d46" distance of L22.start L22.end
  measures "d47" diameter of A14
  measures "d48" diameter of A15
  measures "d49" distance of L23.start L23.end
  measures "d50" distance of P10 P11
  measures "d51" distance of L23.start L25.end
  measures "d52" angle of L23 L25
  measures "d53" distance of L22.end L26.end
  measures "d76" distance of A0.centre P5
  measures "d191" diameter of A23
  measures "d192" diameter of A24
  measures "d193" diameter of A36
  measures "d208" diameter of A41
  measures "d209" diameter of A42
  measures "d218" distance of A9.centre A12.centre
  measures "d219" distance of L33 L34
extrude "Extrude1" add sketch "Sketch1" along normal blind 3 contours A17 | S0 L6 L14 L20 L23 L25 L26 S2 L27 L29 S3 L30 L32 L34 A19 A22 S4 S5 S7 L44 L47 S8 S9 S10 S13 L63 S14 L67 S15 L68 S16 S17 L75 S20 S21 S22 S23 L96 L98 L99 L100 S24 L103 | S2 L63 | S3 S23 L103 | A3 A16 picked at (9.7314, 13.675) makes body 1
ref_plane "WorkPlane1" through (-0.3623, 0.3623, 11) normal (0, 0, 1) x (1, 0, 0)
sketch "Sketch2" plane through (0, 0, 11) normal (0, 0, 1) x (1, 0, 0)
  circle A0 centre (16.2855, -23.3566) radius 1
  circle A1 centre (23.3566, -16.2855) radius 1
  circle A2 centre (-20.3514, 9.3912) radius 1.05
  circle A3 centre (-9.3912, 20.3514) radius 1.05
  line L0 (23.3566, -16.2855) -> (16.2855, -23.3566) construction
  line L1 (16.2855, -23.3566) -> (14.5178, -25.1244) construction
  line L2 (23.3566, -16.2855) -> (25.1244, -14.5178) construction
  line L3 (-23.003, 10.9822) -> (15.1807, -27.2015) construction
  line L4 (15.1807, -27.2015) -> (27.2015, -15.1807) construction
  line L5 (27.2015, -15.1807) -> (-10.9822, 23.003) construction
  line L6 (-10.9822, 23.003) -> (-23.003, 10.9822)
  line L7 (-23.003, 10.9822) -> (-31.1929, 10.9822)
  line L8 (-20.3514, 9.3912) -> (-9.3912, 20.3514) construction
  line L9 (-14.8713, 14.8713) -> (-20.2845, 20.2845) construction
  line L10 (16.2855, -23.3566) -> (18.0533, -25.1244) construction
  line L11 (25.1066, -18.0712) -> (25.1285, -18.0491) construction
  line L12 (0, 0) -> (-3.9112, 3.9112) construction
  line L13 (2.3451, -2.3451) -> (5.0559, 0.3657) construction
  arc A4 (-22.4727, 11.5126) -> (-18.0607, 7.4541) centre (-20.3514, 9.3912) ccw
  arc A5 (-7.4541, 18.0607) -> (-11.5126, 22.4727) centre (-9.3912, 20.3514) ccw
  arc A6 (25.1285, -18.0491) -> (25.1244, -14.5178) centre (23.3566, -16.2855) ccw
  arc A7 (14.5178, -25.1244) -> (18.0533, -25.1244) centre (16.2855, -23.3566) ccw
  line L14 (0, 0) -> (2.3451, -2.3451) construction
  line L15 (-8.5, -12.5) -> (0.2365, -12.5)
  line L16 (12.5, -0.2365) -> (12.5, 8.5)
  line L17 (8.5, 12.5) -> (-0.2365, 12.5)
  line L18 (-12.5, 0.2365) -> (-12.5, -8.5)
  line L19 (-12.5, 12.5) -> (12.5, -12.5) construction
  arc A8 (-12.5, -8.5) -> (-8.5, -12.5) centre (-8.5, -8.5) ccw
  arc A9 (12.5, 8.5) -> (8.5, 12.5) centre (8.5, 8.5) ccw
  line L20 (25.1244, -14.5178) -> (13.6716, -3.065)
  line L21 (-3.065, 13.6716) -> (-7.4541, 18.0607)
  line L22 (14.5178, -25.1244) -> (3.065, -13.6716)
  line L23 (-13.6716, 3.065) -> (-18.0607, 7.4541)
  arc A10 (-12.5, 0.2365) -> (-13.6716, 3.065) centre (-16.5, 0.2365) ccw
  arc A11 (-3.065, 13.6716) -> (-0.2365, 12.5) centre (-0.2365, 16.5) ccw
  arc A12 (12.5, -0.2365) -> (13.6716, -3.065) centre (16.5, -0.2365) ccw
  arc A13 (3.065, -13.6716) -> (0.2365, -12.5) centre (0.2365, -16.5) ccw
  line L24 (0, 0) -> (-15.544, -15.544) construction
  line L25 (18.0533, -25.1244) -> (18.0753, -25.1024)
  line L26 (25.1285, -18.0491) -> (23.7143, -19.4634) construction
  arc A14 (22.4982, -18.6635) -> (18.6635, -22.4982) centre (21.4934, -21.4934) ccw
  arc A15 (22.4982, -18.6635) -> (25.1066, -18.0712) centre (23.3347, -16.3076) ccw
  arc A16 (18.0753, -25.1024) -> (18.6635, -22.4982) centre (16.3075, -23.3346) ccw
  line L27 (0, 0) -> (31.4983, -31.4983) construction
  line L28 (25.1066, -18.0712) -> (25.1285, -18.0491)
  circle A17 centre (-8.4853, -2.8284) radius 1
  circle A18 centre (-2.8284, -8.4853) radius 1
  line L29 (-8.4853, -2.8284) -> (-2.8284, -8.4853) construction
  line L30 (-8.4853, -2.8284) -> (5.3658, -2.8284) construction
  line L31 (-8.4853, -2.8284) -> (-7.7782, -2.1213) construction
  line L32 (-7.7782, -2.1213) -> (-2.1213, -7.7782)
  line L33 (-8.4853, -2.8284) -> (-9.1924, -3.5355) construction
  line L34 (-9.1924, -3.5355) -> (-3.5355, -9.1924)
  line L35 (3.5355, 9.1924) -> (9.1924, 3.5355)
  circle A19 centre (8.4853, 2.8284) radius 1
  line L36 (2.1213, 7.7782) -> (7.7782, 2.1213)
  circle A20 centre (2.8284, 8.4853) radius 1
  point P0 (-14.8713, 14.8713)
  point P1 (-16.9926, 16.9926)
  point P2 (-0.1298, -6.5877)
  point P3 (-12.5, -12.5)
  point P4 (19.4675, -23.7102)
  point P5 (19.37, -19.37)
  point P6 (-5.6569, -5.6569)
  dimension "d57" = 5
  dimension "d58" = 5
  dimension "d59" = 6
  dimension "d60" = 6
  dimension "d63" = 17
  dimension "d64" = 45
  dimension "d65" = 3
  dimension "d91" = 4
  dimension "d92" = 4
  dimension "d93" = 4
  dimension "d94" = 4
  dimension "d95" = 4
  dimension "d115" = 2
  dimension "d116" = 2
  dimension "d117" = 2.5
  dimension "d118" = 2.5
  dimension "d211" = 2
  dimension "d212" = 2
  dimension "d213" = 45
  dimension "d214" = 8
  dimension "d215" = 14
  constraint concentric A0 A7
  constraint concentric A1 A6
  constraint concentric A2 A4
  constraint concentric A3 A5
  constraint coincident A1.centre L0.start
  constraint coincident A0.centre L0.end
  constraint parallel L0 L1
  constraint parallel L0 L2
  constraint perpendicular L3 L4
  constraint parallel L3 L5
  constraint parallel L4 L6
  constraint horizontal L7
  constraint coincident A2.centre L8.start
  constraint coincident A3.centre L8.end
  constraint midpoint L8 P0
  constraint midpoint L6 P1
  constraint coincident P0 L9.start
  constraint perpendicular L6 L9
  constraint coincident P1 L9
  constraint tangent A7 L22
  constraint tangent A6 L20
  constraint perpendicular L1 L10
  constraint tangent L11 A6
  constraint coincident L12.start L14.start
  constraint parallel L12 L20
  constraint perpendicular L12 L13
  constraint coincident L6 A4.start
  constraint coincident L6 A5.end
  constraint perpendicular L13 L14
  constraint coincident L13.start L14.end
  constraint perpendicular L15 L16
  constraint parallel L15 L17
  constraint parallel L16 L18
  constraint midpoint L19 L12.start
  constraint horizontal L17
  constraint coincident P3 L18
  constraint coincident P3 L15
  constraint tangent L18 A8
  constraint tangent L15 A8
  constraint tangent L16 A9
  constraint tangent L17 A9
  constraint collinear L20 L21
  constraint tangent L23 A10
  constraint tangent L18 A10
  constraint tangent L17 A11
  constraint tangent L21 A11
  constraint tangent L20 A12
  constraint tangent L16 A12
  constraint tangent L22 A13
  constraint tangent L15 A13
  constraint perpendicular L14 L24
  constraint tangent A7 L25
  constraint perpendicular L10 L26
  constraint tangent A14 A15
  constraint tangent L11 A15
  constraint coincident P4 L25
  constraint coincident P4 A14
  constraint tangent A14 A16
  constraint tangent L25 A16
  constraint midpoint A14 P5
  constraint perpendicular L24 L27
  constraint coincident P5 L27
  constraint horizontal L30
  constraint coincident A17.centre L29.start
  constraint coincident A18.centre L29.end
  constraint coincident A17 L31.end
  constraint perpendicular L29 L31
  constraint coincident A18 L32.end
  constraint tangent A18 L32
  constraint coincident A17 L33.end
  constraint perpendicular L32 L33
  constraint coincident A18 L34.end
  constraint tangent A18 L34
  constraint symmetric L19 A17 A20
  constraint symmetric L19 A18 A19
  constraint symmetric L19 L31.end L36.start
  constraint symmetric L19 L32.end L36.end
  constraint symmetric L19 L33.end L35.start
  constraint symmetric L19 L34.end L35.end
  constraint midpoint L29 P6
  constraint coincident L24 P6
  measures "d57" diameter of A7
  measures "d58" diameter of A6
  measures "d59" diameter of A4
  measures "d60" diameter of A5
  measures "d63" distance of L3.start L5.end
  measures "d64" angle of L3 L7
  measures "d65" distance of L6 L8
  measures "d91" radius of A9
  measures "d92" radius of A10
  measures "d93" radius of A11
  measures "d94" radius of A12
  measures "d95" radius of A13
  measures "d115" distance of L10.end P4
  measures "d116" distance of L11.end L26.end
  measures "d117" radius of A15
  measures "d118" radius of A16
  measures "d211" diameter of A17
  measures "d212" diameter of A18
  measures "d213" angle of L29 L30
  measures "d214" distance of A17.centre A18.centre
  measures "d215" distance of L32 L36
extrude "Extrusion2" add sketch "Sketch2" along normal blind 2 separate body makes body 2
chamfer "Chamfer2" distance 1 angle 45 4 edges at (-21.3303, 9.7709, 13) (-10.3702, 20.7311, 13) (15.3532, -22.995, 13) (22.4243, -15.9239, 13) on bodies 2
